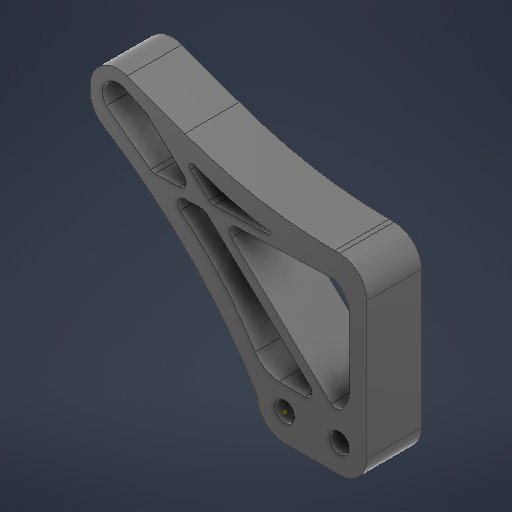
# Autodesk Inventor part: Ring Bay
Saved by Autodesk Inventor 2025 (Build 290162000, 162)
## iProperties
Created: 2024-12-29
Part Number: Ring Bay
Material: Generic
Document SubType Name: Modeling
Designer: Juan
Density: 1 g/cm^3
Appearance: Default
Author: Juan
Autodesk Inventor part; units mm, degrees
ref_plane "YZ Plane" through (0, 0, 0) normal (1, 0, 0) x (0, 1, 0)
ref_plane "XZ Plane" through (0, 0, 0) normal (0, 1, 0) x (-1, 0, 0)
ref_plane "XY Plane" through (0, 0, 0) normal (0, 0, 1) x (1, 0, 0)
sketch "Sketch1" plane through (0, 0, 0) normal (0, 0, 1) x (1, 0, 0)
  circle A0 centre (0, 0) radius 2.3241
  line L0 (0, 0) -> (12.7, 0)
  circle A1 centre (12.7, 0) radius 2.3241
  line L1 (0, 0) -> (12.7, 0) construction
  line L2 (0, -6.35) -> (12.7, -6.35)
  line L3 (12.7, 6.35) -> (0, 6.35)
  arc A2 (0, 6.35) -> (0, -6.35) centre (0, 0) ccw
  arc A3 (12.7, -6.35) -> (12.7, 6.35) centre (12.7, 0) ccw
  point P0 (6.35, 0)
  dimension "d0" = 4.6482
  dimension "d1" = 12.7
  dimension "d2" = 4.6482
  dimension "d3" = 12.7
  constraints: 10 end point, 4 centre point, 4 point on circle, 4 tangent, 2 coincident, 2 horizontal, 1 midpoint, 1 parallel
  measures "d0" diameter of A0
  measures "d1" distance of L0.start L0.end
  measures "d2" diameter of A1
  measures "d3" diameter of A3
extrude "Extrusion1" add sketch "Sketch1" along normal blind 12.7
sketch "Sketch2" plane through (0, 0, 0) normal (0, 0, -1) x (-1, 0, 0)
  circle A0 centre (-12.7, 0) radius 2.3241 projected
  circle A1 centre (0, 0) radius 2.3241 projected
  circle A2 centre (-12.7, 0) radius 4.1275
  circle A3 centre (0, 0) radius 4.1275
  dimension "d6" = 8.255
  dimension "d7" = 8.255
  constraints: 2 centre point, 2 coincident
  measures "d6" diameter of A2
  measures "d7" diameter of A3
extrude "Extrusion2" cut sketch "Sketch2" against normal blind 2.54
sketch "Sketch3" plane through (0, 0, 12.7) normal (0, 0, 1) x (1, 0, 0)
  arc A0 (0, 6.35) -> (0, -6.35) centre (0, 0) ccw projected
  arc A1 (12.7, -6.35) -> (12.7, 6.35) centre (12.7, 0) ccw projected
  line L0 (12.7, 6.35) -> (0, 6.35) projected
  arc A2 (0, 6.35) -> (0, -6.35) centre (0, 0) ccw projected
  line L1 (0, -6.35) -> (12.7, -6.35) projected
  circle A3 centre (0, 0) radius 2.3241 projected
  circle A4 centre (12.7, 0) radius 2.3241 projected
  line L2 (19.05, 0) -> (19.05, 38.1)
  line L3 (-6.35, 0) -> (-6.35, 38.1)
  arc A5 (0, 6.35) -> (0, -6.35) centre (0, 0) ccw projected
  line L4 (-6.35, 38.1) -> (19.05, 38.1)
  line L5 (-6.35, 38.1) -> (-69.85, 38.1)
  line L6 (-6.35, 38.1) -> (-72.261, 62.0897)
  line L7 (-72.261, 62.0897) -> (-72.261, 49.3897)
  arc A6 (-6.35, 0) -> (-72.261, 49.3897) centre (-100.4419, -56.8924) ccw
  line L8 (-34.5064, 31.0993) -> (-34.5064, 48.3481)
  line L9 (-45.0661, 38.1) -> (-45.0661, 52.1915)
  point P0 (0, 6.35)
  point P1 (-34.5064, 38.1)
  dimension "d10" = 38.1
  dimension "d14" = 63.5
  dimension "d15" = 20
  dimension "d16" = 12.7
  constraints: 16 end point, 6 point on circle, 3 perpendicular, 3 point on line, 3 tangent, 3 vertical, 1 centre point, 1 horizontal
  measures "d10" distance of L2.start L2.end
  measures "d14" distance of L3.end L5.end
  measures "d15" angle of L6 L5
  measures "d16" distance of L6.end L7.end
extrude "Extrusion3" add sketch "Sketch3" against normal up to surface (12.7 mm away) contours A0 L3 L4 L2 A1 L0 | A6 L8 L5 L3 | L5 L8 L6
fillet "Fillet1" radius 6.35 1 edges at (19.05, 38.1, 6.35)
fillet "Fillet2" radius 101.6 1 edges at (-6.35, 38.1, 6.35)
extrude "Extrusion7" add sketch "Sketch3" against normal blind 12.7 contours A0 L3 L4 L2 A1 L0 | A6 L8 L5 L3 | A6 L5 L8 | L5 L9 L6 L8
fillet "Fillet3" radius 6.35 3 edges at (-45.0661, 52.1915, 6.35) (-45.0661, 38.1, 6.35) (19.05, 38.1, 6.35)
sketch "Sketch6" plane through (0, 0, 12.7) normal (0, 0, 1) x (1, 0, 0)
  line L0 (-36.5443, 49.0898) -> (-23.1844, 44.2272) projected
  line L1 (-26.9453, 41.2324) -> (-18.0387, 37.9907)
  arc A0 (-23.1844, 44.2272) -> (11.5648, 38.1) centre (11.5648, 139.7) ccw projected
  arc A1 (-18.0387, 37.9907) -> (5.1275, 33.9059) centre (5.1275, 101.6392) ccw
  arc A2 (-36.5443, 49.0898) -> (-45.0661, 43.1228) centre (-38.7161, 43.1228) ccw projected
  arc A3 (-26.9453, 41.2324) -> (-32.6265, 37.2544) centre (-28.3931, 37.2544) ccw
  arc A4 (-45.0661, 41.681) -> (-42.0862, 36.2991) centre (-38.7161, 41.681) ccw projected
  arc A5 (-32.6265, 36.2932) -> (-30.6399, 32.7052) centre (-28.3932, 36.2932) ccw
  line L2 (-45.0661, 41.681) -> (-45.0661, 43.1228) projected
  line L3 (-32.6265, 36.2932) -> (-32.6265, 37.2544)
  arc A6 (-6.35, 0) -> (0, -6.35) centre (0, 0) ccw projected
  arc A7 (-6.8158, 8.5058) -> (-30.6399, 32.7052) centre (-69.5437, -29.4224) ccw
  arc A8 (12.7, -6.35) -> (19.05, 0) centre (12.7, 0) ccw projected
  line L4 (-6.8158, 8.5058) -> (10.1176, 8.5058)
  line L5 (10.1176, 8.5058) -> (10.1176, 30.026)
  line L6 (12.7, 38.1) -> (11.5648, 38.1) projected
  line L7 (5.1275, 33.9059) -> (5.8843, 33.9059)
  arc A9 (10.1176, 30.026) -> (5.8843, 33.9059) centre (5.8784, 29.65) ccw
  circle A10 centre (-38.7161, 43.1228) radius 3.5825
  line L8 (-30.6399, 32.7052) -> (-41.3753, 40.7221)
  line L9 (-37.1542, 46.3469) -> (-25.5432, 40.7221)
  line L10 (-6.8158, 8.5058) -> (-5.0194, 5.3621)
  line L11 (-5.0194, 5.3621) -> (15.0904, 5.3621)
  line L12 (15.0904, 5.3621) -> (15.0904, 31.7435)
  line L13 (15.0904, 31.7435) -> (5.8842, 33.9059)
  point P0 (5.8842, 33.9059)
  constraints: 22 end point, 13 point on circle, 6 centre point, 2 horizontal, 2 parallel, 2 perpendicular, 1 coincident, 1 point on line, 1 tangent, 1 vertical, 1 other
extrude "Extrusion8" cut sketch "Sketch6" against normal blind 12.7 contours A3 L3 A5 L8 A10 L9 L1 | L1 A1 L7 L13 A9 L5 L4 A7 L8 A5 L3 A3 | A10 L8 | L13 L12 L11 L10 L4 L5 A9 picked at (-38.0775, 41.7353)
fillet "Fillet4" radius 6.35 4 edges at (15.0904, 31.7435, 6.35) (5.8842, 33.9059, 6.35) (-5.0194, 5.3621, 6.35) (15.0904, 5.3621, 6.35)
sketch "Sketch7" plane through (0, 0, 12.7) normal (0, 0, 1) x (1, 0, 0)
  point P0 (0, 0)
sketch "Sketch8" plane through (0, 0, 12.7) normal (0, 0, 1) x (1, 0, 0)
  arc A0 (-6.8158, 8.5058) -> (-30.6399, 32.7052) centre (-69.5437, -29.4224) ccw projected
  line L0 (-30.6399, 32.7052) -> (5.4461, 34.0088)
  line L1 (5.4461, 34.0088) -> (12.4378, 32.3666)
  line L2 (10.1924, 32.894) -> (6.6005, 33.7376) projected
  line L3 (12.4378, 32.3666) -> (-28.2224, 30.8977)
  line L4 (-28.2224, 30.8977) -> (-30.6399, 32.7052)
  arc A1 (8.7404, 5.3621) -> (15.0904, 11.7121) centre (8.7404, 11.7121) ccw projected
  line L5 (8.7404, 5.3621) -> (-31.9338, 43.818)
  line L6 (-25.5432, 40.7221) -> (-37.1542, 46.3469) projected
  line L7 (11.702, 6.0501) -> (-26.744, 42.3992)
  line L8 (-26.744, 42.3992) -> (-31.9338, 43.818)
  point P0 (0, 0)
  point P1 (-20.565, 33.0692)
  point P2 (-18.6346, 31.2441)
  point P3 (11.6714, 6.079)
  point P4 (-15.0811, 31.3725)
  point P5 (-17.0115, 33.1975)
  constraints: 14 end point, 2 parallel, 1 collinear, 1 point on line
extrude "Extrusion9" add sketch "Sketch8" against normal blind 12.7
fillet "Fillet5" radius 1.5875 8 edges at (-15.0811, 31.3725, 6.35) (-27.9088, 30.9091, 6.35) (-20.565, 33.0692, 6.35) (-30.6399, 32.7052, 6.35) (8.7404, 5.3621, 6.35) (11.6714, 6.079, 6.35) (-18.6346, 31.2441, 6.35) (-17.0115, 33.1975, 6.35)
fillet "Fillet6" radius 0.7937 1 edges at (-24.6115, 40.383, 6.35)
fillet "Fillet7" radius 0.3969 1 edges at (3.2884, 33.9309, 6.35)
body "Solid1"
